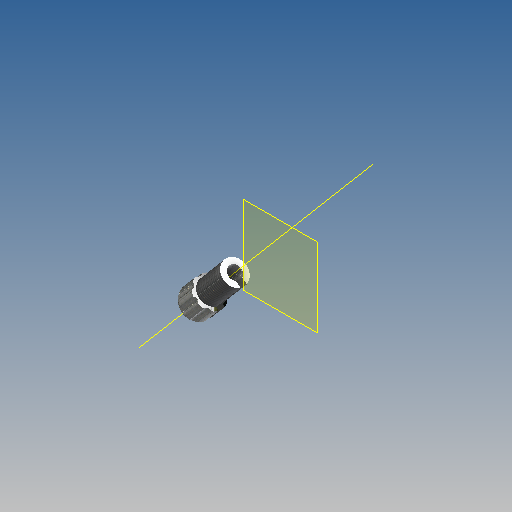
# Autodesk Inventor part: PWTR-0107
Saved by Autodesk Inventor 2021.1 (Build 251245000, 245)
## iProperties
Created: 2015-03-16
Part Number: PWTR-0107
Material: Aluminum 6061
Document SubType Name: Modeling
Designer: baris
Density: 2.7 g/cm^3
Appearance: Aluminum - Flat
Description: Level Adjustment Screw
Author: baris
Revision Number: A
Autodesk Inventor part; units mm, degrees
ref_plane "YZ Plane" through (0, 0, 0) normal (1, 0, 0) x (0, 1, 0)
ref_plane "XZ Plane" through (0, 0, 0) normal (0, 1, 0) x (-1, 0, 0)
ref_plane "XY Plane" through (0, 0, 0) normal (0, 0, 1) x (1, 0, 0)
ref_plane "Work Plane2" through (13.5311, -71.8115, 5) normal (0, 0, 1) x (1, 0, 0)
sketch "Sketch1" plane through (13.5311, -71.8115, 5) normal (0, 0, 1) x (1, 0, 0)
  line L0 (-13.3869, -1.2773) -> (-9.5068, 3.2992)
  line L1 (-13.8304, 0.4097) -> (-20.0134, 5.6518)
  line L2 (10.5341, 27.1106) -> (-13.8304, 0.4097)
  line L3 (-3.5475, 48.261) -> (10.5341, 27.1106)
  line L4 (-3.5475, 48.261) -> (-6.376, 42.0286)
  arc A0 (-4.5989, 24.8494) -> (-6.376, 42.0286) centre (-20.1471, 31.9226) ccw
  line L5 (-4.5989, 24.8494) -> (-12.5466, 7.3787)
  line L6 (-18.0822, 9.8969) -> (-12.5466, 7.3787)
  line L7 (-20.0134, 5.6518) -> (-18.0822, 9.8969)
  line L8 (-8.9114, 15.4215) -> (-12.7915, 10.845)
  line L9 (-10.8515, 13.1333) -> (-5.2184, 8.3574) construction
  line L10 (-8.0349, 10.7453) -> (-29.5854, -14.6732) construction
  line L11 (-9.3702, 5.1499) -> (-18.2298, -5.2999)
  line L12 (-9.3702, 5.1499) -> (-7.6921, 3.7272)
  line L13 (-7.6921, 3.7272) -> (-17.3924, -7.7142)
  line L14 (-17.3924, -7.7142) -> (-16.8141, -8.8876)
  line L15 (-16.8141, -8.8876) -> (-22.0394, -15.0509)
  arc A1 (-24.3119, -15.8757) -> (-22.0394, -15.0509) centre (-23.8969, -13.4761) ccw
  line L16 (-24.3119, -15.8757) -> (-25.456, -14.9056)
  line L17 (-25.456, -14.9056) -> (-19.3125, -7.6594)
  line L18 (-19.3125, -7.6594) -> (-20.8762, -6.3337)
  line L19 (-20.8762, -6.3337) -> (-19.2595, -4.4268)
  line L20 (-19.2595, -4.4268) -> (-18.2298, -5.2999)
  point P0 (-13.5311, 71.8115)
  dimension "d0" = 15
  dimension "d1" = 4.8
  dimension "d2" = 2.6
  dimension "d3" = 6
  dimension "d4" = 10.7
  dimension "d5" = 3.3
  dimension "d6" = 1.25
  dimension "d7" = 2.5
  dimension "d8" = 9.5
  constraints: 42 end point, 8 perpendicular, 4 point on circle, 3 parallel, 2 centre point, 2 midpoint, 2 point on line, 1 tangent, 3 other
  measures "d0" distance from line of L12 L13.end
  measures "d1" distance between parallel lines of L10 L13
  measures "d2" distance between parallel lines of L10 L11
  measures "d3" distance between parallel lines of L10 L15
  measures "d4" distance from line of L16 L13.end
  measures "d5" distance between parallel lines of L10 L17
  measures "d6" distance between parallel lines of L10 L19
  measures "d7" distance between parallel lines of L18 L20
  measures "d8" distance between parallel lines of L16 L18
revolve "Revolution1" add sketch "Sketch1" angle 360 about axis through (5.4962, -61.0662, 5) along (-0.6466853, -0.762757, 0) contours L12 L13 L14 L15 A1 L16 L17 L18 L19 L20 L11
thread "Thread1" size "M10x1" class "6g" standard "ISO Metric profile" full length
sketch "Sketch2" plane through (-14.442, -84.583, 5) normal (-0.6466853, -0.762757, 0) x (0.762757, -0.6466853, 0)
  circle A0 centre (0, 7.0863) radius 1.75
  circle A1 centre (-5.0107, 5.0107) radius 1.75
  circle A2 centre (-7.0863, 0) radius 1.75
  circle A3 centre (-5.0107, -5.0107) radius 1.75
  circle A4 centre (0, -7.0863) radius 1.75
  circle A5 centre (5.0107, -5.0107) radius 1.75
  circle A6 centre (7.0863, 0) radius 1.75
  circle A7 centre (5.0107, 5.0107) radius 1.75
  point P0 (-43.6828, -5)
  point P1 (0, 0)
  point P2 (0, 0)
  point P3 (0, 0)
  point P4 (0, 0)
  point P5 (0, 0)
  point P6 (0, 0)
  point P7 (0, 0)
  point P8 (0, 0)
  point P9 (0, 0)
  dimension "d12" = 3.5
  dimension "d15" = 360
  constraints: 8 centre point, 3 coincident, 23 other
  measures "d12" diameter of A0
extrude "Extrusion1" cut sketch "Sketch2" against normal blind 10.75 contours A0 | A1 | A2 | A3 | A4 | A5 | A7
sketch "Sketch3" plane through (-14.442, -84.583, 5) normal (-0.6466853, -0.762757, 0) x (0.762757, -0.6466853, 0)
  line L0 (0, 0) -> (18.2305, 0) construction
  line L1 (0, 0) -> (0, 1.25)
  line L2 (0, 1.25) -> (6.9946, 1.25)
  line L3 (6.9946, 1.25) -> (6.9946, 0)
  line L4 (0, 0) -> (0, -1.25)
  line L5 (0, -1.25) -> (6.9946, -1.25)
  line L6 (6.9946, -1.25) -> (6.9946, 0)
  point P0 (-43.6828, -5)
  dimension "d19" = 1.25
  constraints: 14 end point, 2 perpendicular, 2 symmetric about line, 1 horizontal, 1 point on line, 1 vertical
  measures "d19" distance between parallel lines of L0 L2
extrude "Extrusion2" cut sketch "Sketch3" against normal through all
body "Solid1"
